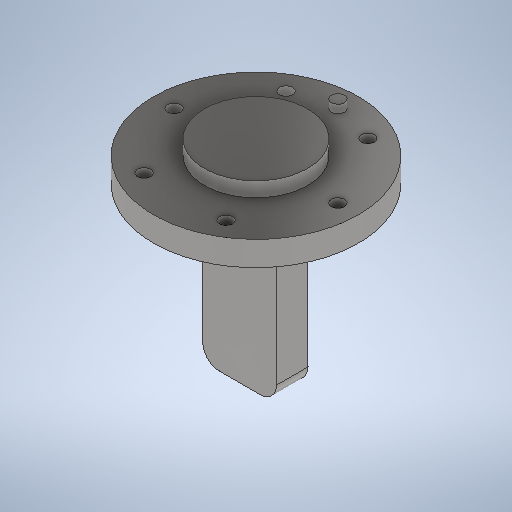
# Autodesk Inventor part: EndEffector
Saved by Autodesk Inventor 2025.1 (Build 291241000, 241)
## iProperties
Created: 2025-01-29
Part Number: EndEffector
Material: Steel, High Strength, Low Alloy
Document SubType Name: Modeling
Designer: yovan
Mass: 4767.32 g
Surface Area: 922.718 cm^2
Volume: 607.302 cm^3
Density: 7.85 g/cm^3
Appearance: Steel - Polished
Author: yovan
Autodesk Inventor part; units mm, degrees
ref_plane "YZ Plane" through (0, 0, 0) normal (1, 0, 0) x (0, 1, 0)
ref_plane "XZ Plane" through (0, 0, 0) normal (0, 1, 0) x (-1, 0, 0)
ref_plane "XY Plane" through (0, 0, 0) normal (0, 0, 1) x (1, 0, 0)
sketch "Sketch3" plane through (0, 0, 0) normal (0, 1, 0) x (-1, 0, 0)
  circle A0 centre (0, 0) radius 62.5
  dimension "d10" = 125
  constraints: 1 centre point, 1 coincident
  measures "d10" diameter of A0
extrude "Extrusion3" add sketch "Sketch3" along normal blind 15
sketch "Sketch6" plane through (0, 0, 0) normal (0, -1, 0) x (1, 0, 0)
  line L0 (22.5, 10) -> (-22.5, 10)
  line L1 (-22.5, 10) -> (-22.5, -10)
  line L2 (-22.5, -10) -> (22.5, -10)
  line L3 (22.5, -10) -> (22.5, 10)
  dimension "d28" = 45
  dimension "d29" = 20
  constraints: 8 end point, 2 parallel, 1 horizontal, 1 perpendicular
  measures "d28" distance of L2.end L1.end
  measures "d29" distance of L1.end L0.end
extrude "Extrusion6" add sketch "Sketch6" along normal blind 100
fillet "Fillet1" radius 10 1 edges at (-22.5, -100, 0)
fillet "Fillet2" radius 10 1 edges at (22.5, -100, 0)
sketch "Sketch8" plane through (22.5, 0, -10) normal (0, 0, -1) x (-1, 0, 0)
  line L0 (22.5, 0) -> (22.5, -40)
  line L1 (22.5, -40) -> (22.5, -75)
  circle A0 centre (22.5, -75) radius 7.5
  circle A1 centre (22.5, -40) radius 7.5
  point P0 (22.5, -32.5)
  point P1 (22.5, -47.5)
  dimension "d37" = 40
  dimension "d38" = 35
  dimension "d39" = 15
  dimension "d40" = 15
  constraints: 4 end point, 2 centre point, 2 coincident, 2 vertical
  measures "d37" distance of L0.start L0.end
  measures "d38" distance of L0.end L1.end
  measures "d39" diameter of A0
  measures "d40" diameter of A1
extrude "Extrusion7" add sketch "Sketch8" along normal blind 10
fillet "Face Fillet1" radius 10 1 edges at (0, 0, -10)
fillet "Fillet3" radius 1 7 edges at (19.5711, -97.0711, -10) (0, -100, -10) (-19.5711, -97.0711, -10) (-22.5, -50, -10) (-22.5, -2.9289, -12.9289) (22.5, -2.9289, -12.9289) (22.5, -50, -10)
sketch "Sketch9" plane through (0, 0, 0) normal (0, -1, 0) x (1, 0, 0)
  circle A0 centre (0, 0) radius 50
  circle A1 centre (-50, 0) radius 4
  circle A2 centre (-25, -43.3013) radius 4
  circle A3 centre (25, -43.3013) radius 4
  circle A4 centre (50, 0) radius 4
  circle A5 centre (25, 43.3013) radius 4
  circle A6 centre (-25, 43.3013) radius 4
  dimension "d45" = 100
  dimension "d46" = 8
  dimension "d49" = 360
  constraints: 6 centre point, 1 horizontal alignment, 15 other
  measures "d46" diameter of A1
extrude "Extrusion8" cut sketch "Sketch9" against normal blind 20 contours A0 A4 | A0 A4 | A5 A0 | A0 A5 | A3 A0 | A0 A3 | A6 A0 | A0 A6 | A2 A0 | A0 A2 | A1 A0 | A0 A1
sketch "Sketch10" plane through (0, 15, 0) normal (0, 1, 0) x (1, 0, 0)
  circle A0 centre (25, 43.3013) radius 4 projected
  circle A1 centre (0, 0) radius 50
  circle A2 centre (0, 50) radius 4
  circle A3 centre (0, 0) radius 31.5
  dimension "d53" = 8
  dimension "d54" = 63
  constraints: 3 centre point, 2 coincident, 2 point on circle
  measures "d53" diameter of A2
  measures "d54" diameter of A3
extrude "Extrusion9" add sketch "Sketch10" along normal blind 9 contours A3
extrude "Extrusion10" add sketch "Sketch10" along normal blind 5 contours A2 A1 | A1 A2
body "Solid2"
